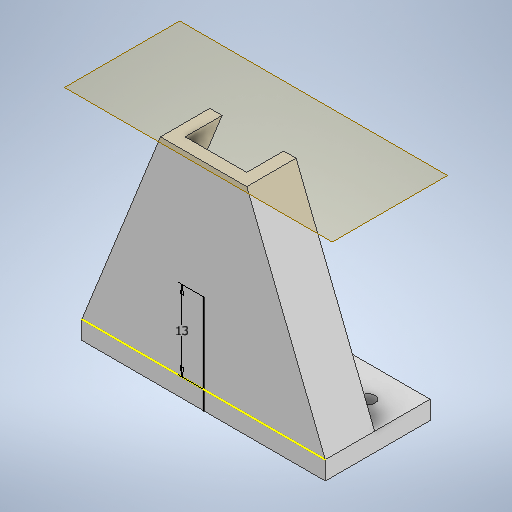
# Autodesk Inventor part: plate
Saved by Autodesk Inventor 2025.1 (Build 291241020, 241B)
## iProperties
Created: 2025-06-05
Part Number: plate
Material: Generic
Document SubType Name: Modeling
Designer: omiye
Density: 1 g/cm^3
Appearance: Default
Author: omiye
Autodesk Inventor part; units mm, degrees
ref_plane "YZ Plane" through (0, 0, 0) normal (1, 0, 0) x (0, 1, 0)
ref_plane "XZ Plane" through (0, 0, 0) normal (0, 1, 0) x (-1, 0, 0)
ref_plane "XY Plane" through (0, 0, 0) normal (0, 0, 1) x (1, 0, 0)
sketch "Sketch1" plane through (0, 0, 0) normal (0, 1, 0) x (-1, 0, 0)
  line L0 (-50, 15) -> (50, 15)
  line L1 (50, 15) -> (50, -15)
  line L2 (50, -15) -> (-50, -15)
  line L3 (-50, -15) -> (-50, 15)
  line L4 (-50, 15) -> (50, -15) construction
  line L5 (50, 15) -> (-50, -15) construction
  point P0 (0, 0)
  dimension "d0" = 100
  dimension "d1" = 30
  constraints: 12 end point, 2 midpoint, 2 parallel, 1 horizontal, 1 perpendicular
  measures "d0" distance of L1.end L2.end
  measures "d1" distance of L0.end L1.end
extrude "Extrusion1" add sketch "Sketch1" along normal blind 3
sketch "Sketch2" plane through (0, 3, 0) normal (0, 1, 0) x (1, 0, 0)
  line L0 (25, -5) -> (-25, -5)
  line L1 (-25, -5) -> (-25, 5)
  line L2 (-25, 5) -> (25, 5)
  line L3 (25, 5) -> (25, -5)
  line L4 (25, -5) -> (-25, 5) construction
  line L5 (-25, -5) -> (25, 5) construction
  line L6 (50, 15) -> (-50, 15) projected
  line L7 (50, -15) -> (-50, -15)
  line L8 (-50, -15) -> (-50, 15)
  line L9 (-50, 15) -> (50, 15)
  line L10 (50, 15) -> (50, -15)
  line L11 (50, -15) -> (-50, 15) construction
  line L12 (-50, -15) -> (50, 15) construction
  point P0 (0, 0)
  dimension "d4" = 50
  dimension "d5" = 10
  constraints: 24 end point, 4 midpoint, 4 parallel, 2 horizontal, 2 perpendicular
  measures "d4" distance of L1.end L2.end
  measures "d5" distance of L0.end L1.end
extrude "Extrusion2" cut sketch "Sketch2" against normal blind 3
sketch "Sketch3" plane through (0, 0, 0) normal (0, -1, 0) x (1, 0, 0)
  line L0 (0, 0) -> (5, 0)
  line L1 (5, 0) -> (-5, 0)
  circle A0 centre (-5, 0) radius 1.1
  circle A1 centre (5, 0) radius 1.1
  line L2 (5, 0) -> (14.75, 0)
  line L3 (-5, 0) -> (-14.75, 0)
  circle A2 centre (14.75, 0) radius 1.1
  circle A3 centre (-14.75, 0) radius 1.1
  dimension "d8" = 5
  dimension "d9" = 10
  dimension "d10" = 2.2
  dimension "d11" = 2.2
  dimension "d12" = 9.75
  dimension "d13" = 9.75
  dimension "d14" = 2.2
  dimension "d15" = 2.2
  constraints: 8 end point, 4 centre point, 4 coincident, 2 horizontal, 2 point on line
  measures "d8" distance of L0.start L0.end
  measures "d9" distance of L0.end L1.end
  measures "d10" diameter of A0
  measures "d11" diameter of A1
  measures "d12" distance of L2.start L2.end
  measures "d13" distance of L3.start L3.end
  measures "d14" diameter of A2
  measures "d15" diameter of A3
extrude "Extrusion3" cut sketch "Sketch3" against normal blind 3.95
sketch "Sketch4" plane through (0, 3, 0) normal (0, 1, 0) x (1, 0, 0)
  circle A0 centre (-14.75, 0) radius 1.1 projected
  line L0 (-14.75, 0) -> (-19.75, 0)
  line L1 (-19.75, 0) -> (-19.75, 5)
  line L2 (25, 5) -> (-25, 5) projected
  line L3 (-19.75, 0) -> (-19.75, -5)
  line L4 (-25, -5) -> (25, -5) projected
  circle A1 centre (14.75, 0) radius 1.1 projected
  line L5 (14.75, 0) -> (19.75, 0)
  line L6 (19.75, 0) -> (19.75, 5.4669)
  line L7 (19.75, 5.4669) -> (19.75, -5)
  line L8 (-25, 5) -> (-19.75, 5)
  line L9 (-19.75, 5) -> (-19.75, -5)
  line L10 (-19.75, -5) -> (-25, -5)
  line L11 (-25, -5) -> (-25, 5)
  line L12 (19.75, -5) -> (25, -5)
  line L13 (25, -5) -> (25, 5)
  line L14 (25, 5) -> (19.75, 5)
  line L15 (19.75, 5) -> (19.75, -5)
  point P0 (0, 0)
  dimension "d18" = 5
  dimension "d19" = 5
  constraints: 28 end point, 5 point on line, 4 parallel, 4 perpendicular, 3 horizontal
  measures "d18" distance of L0.start L0.end
  measures "d19" distance of L5.start L5.end
extrude "Extrusion4" cut sketch "Sketch4" against normal blind 3.95 contours L3 L4 L11 L2 L1 | L2 L13 L4 L7 L6
sketch "Sketch5" plane through (0, 3, 0) normal (0, 1, 0) x (1, 0, 0)
  circle A0 centre (-14.75, 0) radius 1.1 projected
  line L0 (-14.75, 0) -> (-14.75, -12)
  line L1 (-19.75, -5) -> (19.75, -5) projected
  line L2 (-14.75, 0) -> (-2.75, 0) construction
  line L3 (-14.75, -12) -> (14.75, -12)
  circle A1 centre (14.75, 0) radius 1.1 projected
  line L4 (14.75, -12) -> (14.75, 0)
  line L5 (14.75, 0) -> (-14.75, 0)
  line L6 (-14.75, -12) -> (14.75, -12)
  line L7 (14.75, -12) -> (14.75, -10)
  line L8 (14.75, -10) -> (-14.75, -10)
  line L9 (-14.75, -10) -> (-14.75, -12)
  line L10 (2.5, -24) -> (-2.5, -24)
  line L11 (-2.5, -24) -> (-2.5, 0)
  line L12 (-2.5, 0) -> (2.5, 0)
  line L13 (2.5, 0) -> (2.5, -24)
  line L14 (2.5, -24) -> (-2.5, 0) construction
  line L15 (-2.5, -24) -> (2.5, 0) construction
  line L16 (-14.75, -12) -> (-19.75, -12)
  line L17 (-19.75, -12) -> (-19.75, -5)
  line L18 (-19.75, -5) -> (-14.75, -5)
  line L19 (-14.75, -5) -> (-14.75, -12)
  line L20 (14.75, -12) -> (19.75, -12)
  line L21 (19.75, -12) -> (19.75, -5)
  line L22 (19.75, -5) -> (14.75, -5)
  line L23 (14.75, -5) -> (14.75, -12)
  point P0 (0, 0)
  point P1 (0, -12)
  point P2 (2.5, -5)
  point P3 (2.5, -10)
  point P4 (-2.5, -10)
  point P5 (-2.5, -5)
  dimension "d22" = 12
  dimension "d23" = 90
  dimension "d24" = 2
  dimension "d25" = 5
  constraints: 46 end point, 9 perpendicular, 8 parallel, 4 horizontal, 3 midpoint, 1 point on line
  measures "d22" distance of L0.start L0.end
  measures "d23" angle of L0 L2
  measures "d24" distance of L7.end L6.end
  measures "d25" distance of L10.start L10.end
extrude "Extrusion5" add sketch "Sketch5" against normal up to surface (3 mm away) contours L1 L11 L8 L0 | L0 L16 L17 L1 | L8 L11 L3 L0 | L1 L4 L8 L13 | L8 L13 L3 L11 | L1 L21 L20 L4 | L8 L4 L3 L13
sketch "Sketch6" plane through (0, 3, 0) normal (0, 1, 0) x (1, 0, 0)
  line L0 (-19.75, -12) -> (-19.75, 5) projected
  line L1 (19.75, 5) -> (19.75, -12) projected
  line L2 (-19.75, -12) -> (19.75, -12)
  line L3 (19.75, -12) -> (19.75, -10)
  line L4 (19.75, -10) -> (-19.75, -10)
  line L5 (-19.75, -10) -> (-19.75, -12)
  point P0 (0, 0)
  dimension "d28" = 2
  constraints: 8 end point, 2 parallel, 1 horizontal, 1 perpendicular, 1 point on line
  measures "d28" distance of L3.end L2.end
ref_plane "Work Plane1" through (0, 35, 0) normal (0, 1, 0) x (1, 0, 0)
sketch "Sketch7" plane through (0, 35, 0) normal (0, 1, 0) x (1, 0, 0)
  line L0 (7, -14) -> (-7, -14)
  line L1 (-7, -14) -> (-7, -10)
  line L2 (-7, -10) -> (7, -10)
  line L3 (7, -10) -> (7, -14)
  line L4 (-19.75, -12) -> (19.75, -12) projected
  line L5 (7, -14) -> (-7, -10) construction
  line L6 (-7, -14) -> (7, -10) construction
  line L7 (-7, -12) -> (7, -12)
  point P0 (0, 0)
  point P1 (0, -12)
  dimension "d30" = 14
  constraints: 14 end point, 5 midpoint, 2 parallel, 2 point on line, 1 perpendicular
  measures "d30" distance of L0.start L0.end
loft "Loft1" add profiles "Sketch6", "Sketch7" contours all / L4 L1 L2 L3
sketch "Sketch8" plane through (2.5, 0, 10) normal (0, 0, -1) x (-1, 0, 0)
  line L0 (22.25, 0) -> (22.25, 3) projected
  line L1 (-4.5, 35) -> (9.5, 35) projected
  line L2 (22.25, 3) -> (9.5, 35)
  line L3 (9.5, 35) -> (7.5, 35)
  line L4 (-17.25, 3) -> (22.25, 3) projected
  line L5 (22.25, 3) -> (20.25, 3)
  line L6 (20.25, 3) -> (7.5, 35)
  line L7 (-4.5, 35) -> (-2.5, 35)
  line L8 (-17.25, 3) -> (-4.5, 35) projected
  line L9 (-17.25, 3) -> (-15.25, 3)
  line L10 (-15.25, 3) -> (-2.5, 35)
  line L11 (-4.5, 35) -> (-17.25, 3)
  point P0 (2.5, 0)
  dimension "d35" = 2
  dimension "d36" = 2
  dimension "d37" = 2
  dimension "d38" = 2
  constraints: 16 end point, 3 point on line, 1 horizontal
  measures "d35" distance of L1.end L3.end
  measures "d36" distance of L0.end L5.end
  measures "d37" distance of L1.start L7.end
  measures "d38" distance of L4.start L9.end
extrude "Extrusion6" add sketch "Sketch8" along normal blind 6 contours L1 L10 L4 L8 | L1 L2 L4 L6
sketch "Sketch9" plane through (-19.75, 0, 12) normal (0, 0, 1) x (1, 0, 0)
  line L0 (39.5, 3) -> (0, 3) projected
  line L1 (0, 3) -> (39.5, 3)
  line L2 (19.75, 0) -> (19.75, 3)
  line L3 (19.75, 3) -> (19.75, 16)
  dimension "d41" = 13
  constraints: 6 end point, 1 collinear, 1 midpoint, 1 point on line
  measures "d41" distance of L2.end L3.end
body "Solid1"
